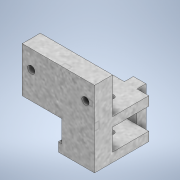
# Autodesk Inventor part: Soporte Idler Z
Saved by Autodesk Inventor 2021 (Build 250183000, 183)
## iProperties
Created: 2023-01-20
Part Number: Soporte Idler Z
Material: Hormigón reforzado con fibra de vidrio
Document SubType Name: Modeling
Designer: Diego.labarca
Density: 1.7 g/cm^3
Appearance: Plano - Pulido Gris
Author: Diego.labarca
Autodesk Inventor part; units mm, degrees
ref_plane "YZ Plane" through (0, 0, 0) normal (1, 0, 0) x (0, 1, 0)
ref_plane "XZ Plane" through (0, 0, 0) normal (0, 1, 0) x (-1, 0, 0)
ref_plane "XY Plane" through (0, 0, 0) normal (0, 0, 1) x (1, 0, 0)
sketch "Boceto1" plane through (0, 0, 0) normal (0, 0, 1) x (1, 0, 0)
  line L0 (-20, 10) -> (20, 10)
  line L1 (20, 10) -> (20, -10)
  line L2 (20, -10) -> (-20, -10)
  line L3 (-20, -10) -> (-20, 10)
  line L4 (0, 0) -> (0, 1.7227)
  line L5 (0, 0) -> (-2.1619, 0)
  line L6 (20, -10) -> (2, -10)
  line L7 (2, -10) -> (2, -27)
  line L8 (2, -27) -> (20, -27)
  line L9 (20, -27) -> (20, -10)
  circle A0 centre (15, 0) radius 2
  circle A1 centre (-15, 0) radius 2
  dimension "d14" = 40
  dimension "d15" = 20
  dimension "d16" = 18
  dimension "d17" = 17
  dimension "d18" = 4
  dimension "d19" = 4
  dimension "d20" = 5
  dimension "d21" = 5
  constraints: 20 end point, 4 parallel, 3 horizontal, 2 centre point, 2 perpendicular, 1 vertical, 2 other
  measures "d14" distance of L1.end L2.end
  measures "d15" distance of L0.end L1.end
  measures "d16" distance of L8.end L7.end
  measures "d17" distance of L7.end L6.end
  measures "d18" diameter of A0
  measures "d19" diameter of A1
  measures "d20" distance from line of A0.centre L1
  measures "d21" distance from line of L3 A1.centre
extrude "Extrusión1" add sketch "Boceto1" along normal blind 10
sketch "Boceto2" plane through (2, -27, 0) normal (0, -1, 0) x (1, 0, 0)
  line L0 (18, 10) -> (-22, 10) projected
  line L1 (18, 10) -> (-2, 10)
  line L2 (-2, 10) -> (-2, -20)
  line L3 (-2, -20) -> (18, -20)
  line L4 (18, -20) -> (18, 10)
  point P0 (-2, 0)
  point P1 (-2, 10)
  dimension "d22" = 30
  dimension "d53" = 20
  constraints: 8 end point, 2 parallel, 1 horizontal, 1 perpendicular
  measures "d22" distance of L2.end L1.end
  measures "d53" distance of L2.end L3.end
extrude "Extrusión2" add sketch "Boceto2" along normal blind 5
sketch "Boceto4" plane through (-20, -10, 0) normal (-1, 0, 0) x (0, 0, 1)
  line L0 (0, 0) -> (0, -17) projected
  line L1 (10, 20) -> (10, 0) projected
  line L2 (10, 0) -> (-20, 0)
  line L3 (-20, 0) -> (-20, -5)
  line L4 (-20, -5) -> (10, -5)
  line L5 (10, -5) -> (10, 0)
  line L6 (10, -22) -> (-20, -22) projected
  point P0 (0, 10)
  dimension "d32" = 5
  dimension "d43" = 30
  dimension "d44" = 30
  constraints: 8 end point, 2 parallel, 1 horizontal, 1 perpendicular
  measures "d32" distance of L3.end L2.end
  measures "d43" distance of L6.start L6.end
  measures "d44" distance of L3.end L4.end
extrude "Extrusión4" add sketch "Boceto4" against normal up to surface (40 mm away)
sketch "Boceto5" plane through (2, -32, 0) normal (0, -1, 0) x (1, 0, 0)
  circle A0 centre (8, -9) radius 1.75
  line L0 (18, -20) -> (18, 10) projected
  circle A1 centre (-17, -9) radius 1.75
  line L1 (-2, -20) -> (18, -20) projected
  line L2 (-22, -20) -> (18, -20) projected
  line L3 (-22, -20) -> (-22, 10) projected
  line L4 (-22, 0) -> (18, 0) projected
  point P0 (-2, 0)
  point P1 (0, 0)
  dimension "d33" = 3.5
  dimension "d34" = 10
  dimension "d37" = 3.5
  dimension "d38" = 5
  dimension "d41" = 9
  dimension "d42" = 9
  constraints: 2 centre point
  measures "d33" diameter of A0
  measures "d34" distance from line of L0 A0.centre
  measures "d37" diameter of A1
  measures "d38" distance from line of L3 A1.centre
  measures "d41" vertical distance of A0.centre point (0, 0)
  measures "d42" distance from line of L4 A1.centre
extrude "Extrusión5" cut sketch "Boceto5" against normal up to surface (22 mm away) contours A0 | A1
sketch "Boceto7" plane through (20, -27, -20) normal (0, 0, -1) x (-1, 0, 0)
  line L0 (0, -5) -> (20, -5) projected
  line L1 (40, 17) -> (0, 17) projected
  line L2 (10, -5) -> (10, -5.3641)
  line L3 (13.5, -5) -> (13.5, 17)
  line L4 (6.5, -5) -> (6.5, 17)
  point P0 (20, 27)
  dimension "d47" = 7
  constraints: 6 end point, 4 point on line, 2 perpendicular, 1 midpoint, 1 vertical, 1 other
  measures "d47" distance between parallel lines of L4 L3
extrude "Extrusión7" add sketch "Boceto7" along normal blind 5
equation "\"d19\" = d18"
equation "\"d21\" = d20"
equation "\"d44\" = d43"
equation "\"d37\" = d33"
